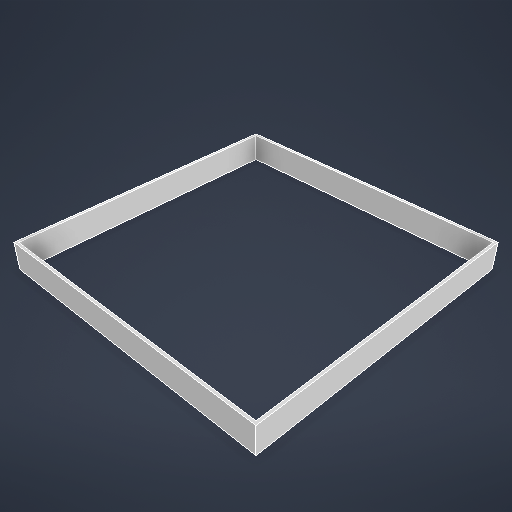
# Autodesk Inventor part: Game_Mat_Inner_Wall
Saved by Autodesk Inventor 2025 (Build 290162000, 162)
## iProperties
Created: 2024-07-08
Part Number: Game_Mat_Inner_Wall
Material: Generic
Document SubType Name: Modeling
Designer: Garfieldcmix
Density: 1 g/cm^3
Appearance: Default
Author: Garfieldcmix
Autodesk Inventor part; units mm, degrees
ref_plane "YZ Plane" through (0, 0, 0) normal (1, 0, 0) x (0, 1, 0)
ref_plane "XZ Plane" through (0, 0, 0) normal (0, 1, 0) x (-1, 0, 0)
ref_plane "XY Plane" through (0, 0, 0) normal (0, 0, 1) x (1, 0, 0)
sketch "Sketch1" plane through (0, 0, 0) normal (0, 1, 0) x (-1, 0, 0)
  line L0 (0, 0) -> (1020, 0)
  line L1 (1020, 0) -> (1020, -1020)
  line L2 (1020, -1020) -> (0, -1020)
  line L3 (0, -1020) -> (0, 0)
  line L4 (1020, -510) -> (0, -510) construction
  line L5 (10, -10) -> (1010, -10)
  line L6 (1010, -10) -> (1010, -1010)
  line L7 (1010, -1010) -> (10, -1010)
  line L8 (10, -1010) -> (10, -10)
  line L9 (1010, -510) -> (10, -510) construction
  point P0 (510, -510)
  dimension "d0" = 1020
  dimension "d1" = 1020
  dimension "d2" = 1000
  dimension "d3" = 1000
  constraints: 20 end point, 6 midpoint, 4 parallel, 2 horizontal, 2 perpendicular
  measures "d0" distance of L1.end L2.end
  measures "d1" distance of L0.end L1.end
  measures "d2" distance of L6.end L7.end
  measures "d3" distance of L5.end L6.end
extrude "Extrusion1" add sketch "Sketch1" along normal blind 100
body "Solid1"
